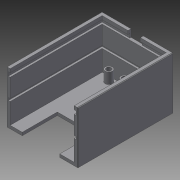
# Autodesk Inventor part: TOP
Saved by Autodesk Inventor 2014 SP1 (Build 180222100, 222)
## iProperties
Created: 2013-12-02
Part Number: TOP
Material: Generic
Document SubType Name: Modeling
Designer: Dominik
Density: 1 g/cm^3
Appearance: Default
Author: Dominik
Autodesk Inventor part; units mm, degrees
ref_plane "YZ Plane" through (0, 0, 0) normal (1, 0, 0) x (0, 1, 0)
ref_plane "XZ Plane" through (0, 0, 0) normal (0, 1, 0) x (-1, 0, 0)
ref_plane "XY Plane" through (0, 0, 0) normal (0, 0, 1) x (1, 0, 0)
sketch "Sketch1" plane through (0, 0, 0) normal (0, 0, 1) x (1, 0, 0)
  line L0 (0, 0) -> (59, 0)
  line L1 (59, 0) -> (59, 79)
  line L2 (59, 79) -> (0, 79)
  line L3 (0, 79) -> (0, 0)
  dimension "d0" = 59
  dimension "d1" = 79
  constraints: 8 end point, 1 horizontal, 1 vertical
  measures "d0" distance between parallel lines of L1 L3
  measures "d1" distance between parallel lines of L2 L0
extrude "Extrusion1" add sketch "Sketch1" along normal blind 3
sketch "Sketch2" plane through (0, 0, 3) normal (0, 0, 1) x (1, 0, 0)
  line L0 (59, 0) -> (59, 79) projected
  line L1 (0, 79) -> (0, 0) projected
  line L2 (0, 0) -> (0, 79) projected
  line L3 (0, 79) -> (59, 79) projected
  line L4 (59, 79) -> (59, 0) projected
  line L5 (59, 0) -> (0, 0) projected
  line L6 (3, 0) -> (56, 0)
  line L7 (56, 0) -> (56, 76)
  line L8 (56, 76) -> (3, 76)
  line L9 (3, 76) -> (3, 0)
  dimension "d25" = 3
  dimension "d26" = 3
  dimension "d27" = 3
  constraints: 8 end point, 1 point on line
  measures "d25" distance between parallel lines of L3 L8
  measures "d26" distance between parallel lines of L0 L7
  measures "d27" distance between parallel lines of L1 L9
extrude "Extrusion2" add sketch "Sketch2" along normal blind 40.5 contours L5 L7 L8 L9 L1 L3 L0
sketch "Sketch3" plane through (0, 0, 0) normal (0, 0, -1) x (-1, 0, 0)
  line L0 (0, 0) -> (-59, 0) projected
  line L1 (0, 79) -> (0, 0) projected
  line L2 (-59, 79) -> (0, 79) projected
  line L3 (-59, 0) -> (-59, 79) projected
  line L4 (-3, 76) -> (-3, 3) construction
  line L5 (-3, 3) -> (-56, 3) construction
  line L6 (-56, 3) -> (-56, 76) construction
  line L7 (-56, 76) -> (-3, 76) construction
  line L8 (-3, 76) -> (-56, 76) construction
  line L9 (-56, 76) -> (-56, 75) construction
  line L10 (-56, 75) -> (-3, 75) construction
  line L11 (-3, 75) -> (-3, 76) construction
  line L12 (-3, 75) -> (-9.5, 75) construction
  line L13 (-9.5, 75) -> (-9.5, 69) construction
  line L14 (-9.5, 69) -> (-3, 69) construction
  line L15 (-3, 69) -> (-3, 75) construction
  line L16 (-9.5, 69) -> (-15.5, 69) construction
  line L17 (-15.5, 69) -> (-15.5, 75) construction
  line L18 (-15.5, 75) -> (-9.5, 75) construction
  line L19 (-9.5, 75) -> (-9.5, 69) construction
  line L20 (-3, 69) -> (-22.5, 69) construction
  line L21 (-22.5, 69) -> (-22.5, 75) construction
  line L22 (-22.5, 75) -> (-3, 75) construction
  line L23 (-3, 75) -> (-3, 69) construction
  line L24 (-22.5, 69) -> (-28.5, 69) construction
  line L25 (-28.5, 69) -> (-28.5, 75) construction
  line L26 (-28.5, 75) -> (-22.5, 75) construction
  line L27 (-22.5, 75) -> (-22.5, 69) construction
  line L28 (-3, 69) -> (-35.5, 69) construction
  line L29 (-35.5, 69) -> (-35.5, 75) construction
  line L30 (-35.5, 75) -> (-3, 75) construction
  line L31 (-3, 75) -> (-3, 69) construction
  line L32 (-35.5, 69) -> (-41.5, 69) construction
  line L33 (-41.5, 69) -> (-41.5, 75) construction
  line L34 (-41.5, 75) -> (-35.5, 75) construction
  line L35 (-35.5, 75) -> (-35.5, 69) construction
  line L36 (-9.5, 69) -> (-15.5, 75) construction
  line L37 (-15.5, 69) -> (-9.5, 75) construction
  line L38 (-22.5, 69) -> (-28.5, 75) construction
  line L39 (-28.5, 69) -> (-22.5, 75) construction
  line L40 (-35.5, 69) -> (-41.5, 75) construction
  line L41 (-41.5, 69) -> (-35.5, 75) construction
  circle A0 centre (-12.5, 72) radius 3
  circle A1 centre (-25.5, 72) radius 3
  circle A2 centre (-38.5, 72) radius 3
  circle A3 centre (-12.5, 72) radius 2
  circle A4 centre (-25.5, 72) radius 2
  circle A5 centre (-38.5, 72) radius 2
  dimension "d9" = 3
  dimension "d10" = 1
  dimension "d11" = 6.5
  dimension "d12" = 6
  dimension "d13" = 6
  dimension "d14" = 19.5
  dimension "d15" = 6
  dimension "d16" = 32.5
  dimension "d17" = 6
  dimension "d18" = 1
  dimension "d19" = 1
  dimension "d20" = 1
  constraints: 76 end point, 6 centre point, 6 point on line, 5 horizontal, 5 vertical, 4 tangent, 3 coincident, 3 midpoint, 3 other
  measures "d9" distance between parallel lines of L2 L7
  measures "d10" distance between parallel lines of L8 L10
  measures "d11" distance between parallel lines of L15 L13
  measures "d12" distance between parallel lines of L12 L14
  measures "d13" distance between parallel lines of L17 L19
  measures "d14" distance between parallel lines of L21 L23
  measures "d15" distance between parallel lines of L25 L27
  measures "d16" distance between parallel lines of L29 L31
  measures "d17" distance between parallel lines of L33 L35
  measures "d18" radial gap between concentric circles of A0 A3
  measures "d19" radial gap between concentric circles of A1 A4
  measures "d20" radial gap between concentric circles of A2 A5
extrude "Extrusion3" add sketch "Sketch3" against normal blind 12 contours A0 | A1 | A2
sketch "Sketch4" plane through (12.5, 72, 3) normal (0, 0, 1) x (1, 0, 0)
  circle A0 centre (0, 0) radius 2 projected
  circle A1 centre (0, 0) radius 2
  circle A2 centre (26, 0) radius 2 projected
  circle A3 centre (26, 0) radius 3 projected
  circle A4 centre (0, 0) radius 2 projected
  circle A5 centre (0, 0) radius 3 projected
  circle A6 centre (13, 0) radius 2 projected
  circle A7 centre (13, 0) radius 3 projected
  circle A8 centre (13, 0) radius 2
  circle A9 centre (26, 0) radius 2
  line L0 (-12.5, -72) -> (-12.5, 7) projected
  line L1 (-12.5, 7) -> (46.5, 7) projected
  line L2 (46.5, 7) -> (46.5, -72) projected
  line L3 (46.5, -72) -> (43.5, -72) projected
  line L4 (43.5, -72) -> (-9.5, -72) projected
  line L5 (-9.5, -72) -> (-12.5, -72) projected
  line L6 (43.5, -72) -> (43.5, 4) projected
  line L7 (43.5, 4) -> (-9.5, 4) projected
  line L8 (-9.5, 4) -> (-9.5, -72) projected
  constraints: 3 centre point, 3 coincident
extrude "Extrusion4" cut sketch "Sketch4" against normal up to next contours A0 | A2 | A6
sketch "Sketch5" plane through (56, 0, 3) normal (-1, 0, 0) x (0, 0, 1)
  line L0 (40.5, 0) -> (0, 0) projected
  line L1 (0, 76) -> (40.5, 76) projected
  line L2 (0, 76) -> (17, 76) construction
  line L3 (17, 76) -> (17, 0) construction
  line L4 (17, 0) -> (0, 0) construction
  line L5 (0, 0) -> (0, 76) construction
  line L6 (17, 0) -> (19.2, 0)
  line L7 (19.2, 0) -> (19.2, 76)
  line L8 (19.2, 76) -> (17, 76)
  line L9 (17, 76) -> (17, 0)
  point P0 (-3, 0)
  dimension "d28" = 17
  dimension "d29" = 2.2
  constraints: 16 end point, 2 point on line
  measures "d28" distance between parallel lines of L5 L3
  measures "d29" distance between parallel lines of L9 L7
extrude "Extrusion5" cut sketch "Sketch5" against normal blind 1.5
sketch "Sketch8" plane through (3, 76, 3) normal (0, -1, 0) x (1, 0, 0)
  line L0 (0, 0) -> (0, 40.5) projected
  line L1 (54.5, 19.2) -> (0, 19.2)
  line L2 (0, 19.2) -> (0, 17)
  line L3 (0, 17) -> (54.5, 17)
  line L4 (54.5, 17) -> (54.5, 19.2)
  point P0 (-3, -3)
  constraints: 8 end point, 1 point on line
extrude "Extrusion8" cut sketch "Sketch8" against normal blind 1.5
sketch "Sketch9" plane through (3, 0, 3) normal (1, 0, 0) x (0, 0, -1)
  line L0 (0, 0) -> (-40.5, 0) projected
  line L1 (-19.2, 77.5) -> (-17, 77.5)
  line L2 (-17, 77.5) -> (-17, 0)
  line L3 (-17, 0) -> (-19.2, 0)
  line L4 (-19.2, 0) -> (-19.2, 77.5)
  point P0 (3, 0)
  constraints: 8 end point, 1 point on line
extrude "Extrusion9" cut sketch "Sketch9" against normal blind 1.5
sketch "Sketch10" plane through (56, 0, 43.5) normal (-1, 0, 0) x (0, 0, 1)
  line L0 (0, 0) -> (-21.3, 0) projected
  line L1 (-21.3, 76) -> (0, 76) projected
  line L2 (0, 0) -> (-2.9, 0) construction
  line L3 (-2.9, 0) -> (-2.9, 76) construction
  line L4 (-2.9, 76) -> (0, 76) construction
  line L5 (0, 76) -> (0, 0) construction
  line L6 (-2.9, 76) -> (-6.1, 76)
  line L7 (-6.1, 76) -> (-6.1, 0)
  line L8 (-6.1, 0) -> (-2.9, 0)
  line L9 (-2.9, 0) -> (-2.9, 76)
  point P0 (-43.5, 0)
  dimension "d40" = 2.9
  dimension "d41" = 3.2
  constraints: 16 end point, 2 point on line
  measures "d40" distance between parallel lines of L3 L5
  measures "d41" distance between parallel lines of L7 L9
extrude "Extrusion10" cut sketch "Sketch10" against normal blind 1.5
sketch "Sketch11" plane through (3, 76, 43.5) normal (0, -1, 0) x (1, 0, 0)
  line L0 (0, -21.3) -> (0, 0) projected
  line L1 (54.5, -2.9) -> (0, -2.9)
  line L2 (0, -2.9) -> (0, -6.1)
  line L3 (0, -6.1) -> (54.5, -6.1)
  line L4 (54.5, -6.1) -> (54.5, -2.9)
  point P0 (-3, -43.5)
  constraints: 8 end point, 1 point on line
extrude "Extrusion11" cut sketch "Sketch11" against normal blind 1.5
sketch "Sketch12" plane through (3, 0, 43.5) normal (1, 0, 0) x (0, 0, -1)
  line L0 (21.3, 0) -> (0, 0) projected
  line L1 (6.1, 77.5) -> (2.9, 77.5)
  line L2 (2.9, 77.5) -> (2.9, 0)
  line L3 (2.9, 0) -> (6.1, 0)
  line L4 (6.1, 0) -> (6.1, 77.5)
  point P0 (43.5, 0)
  constraints: 8 end point, 1 point on line
extrude "Extrusion12" cut sketch "Sketch12" against normal blind 1.5
sketch "Sketch13" plane through (0, 0, 43.5) normal (0, 0, 1) x (1, 0, 0)
  line L0 (3, 76) -> (56, 76) projected
  line L1 (59, 0) -> (59, 79) projected
  line L2 (59, 79) -> (0, 79) projected
  line L3 (0, 79) -> (24.4, 79) construction
  line L4 (24.4, 79) -> (24.4, 76) construction
  line L5 (24.4, 76) -> (0, 76) construction
  line L6 (0, 76) -> (0, 79) construction
  line L7 (34.6, 79) -> (59, 79) construction
  line L8 (59, 79) -> (59, 76) construction
  line L9 (59, 76) -> (34.6, 76) construction
  line L10 (34.6, 76) -> (34.6, 79) construction
  line L11 (24.4, 79) -> (34.6, 79)
  line L12 (34.6, 79) -> (34.6, 76)
  line L13 (34.6, 76) -> (24.4, 76)
  line L14 (24.4, 76) -> (24.4, 79)
  dimension "d48" = 24.4
  dimension "d49" = 24.4
  dimension "d50" = 10.2
  constraints: 24 end point, 3 point on line
  measures "d48" distance between parallel lines of L6 L4
  measures "d49" distance between parallel lines of L1 L10
  measures "d50" distance between parallel lines of L10 L4
extrude "Extrusion13" cut sketch "Sketch13" against normal blind 6.1
sketch "Sketch14" plane through (0, 0, 3) normal (0, 0, 1) x (1, 0, 0)
  line L0 (56, 0) -> (56, 76) projected
  line L1 (3, 76) -> (3, 0) projected
  line L2 (3, 0) -> (56, 0) projected
  line L3 (3, 0) -> (13, 0) construction
  line L4 (13, 0) -> (13, 29) construction
  line L5 (13, 29) -> (3, 29) construction
  line L6 (3, 29) -> (3, 0) construction
  line L7 (13, 29) -> (44, 29)
  line L8 (44, 29) -> (44, 0)
  line L9 (44, 0) -> (13, 0)
  line L10 (13, 0) -> (13, 29)
  point P0 (0, 0)
  dimension "d53" = 29
  dimension "d54" = 10
  dimension "d55" = 12
  constraints: 16 end point, 1 point on line
  measures "d53" distance between parallel lines of L3 L5
  measures "d54" distance between parallel lines of L1 L4
  measures "d55" distance between parallel lines of L0 L8
extrude "Extrusion14" cut sketch "Sketch14" against normal up to next
chamfer "Chamfer1" distance 0.5 angle 45 19 edges at (46.8, 79, 43.5) (59, 39.5, 43.5) (12.2, 79, 43.5) (0, 39.5, 43.5) (0, 0, 21.75) (6.5, 0, 0) (51.5, 0, 0) (59, 0, 21.75) (59, 39.5, 0) (0, 39.5, 0) (29.5, 79, 0) (10.5, 72, 0) (23.5, 72, 0) (36.5, 72, 0) (59, 79, 21.75) (0, 79, 21.75) (24.4, 79, 40.45) (29.5, 79, 37.4) (34.6, 79, 40.45)
chamfer "Chamfer2" distance 0.5 angle 45 3 edges at (13, 14.75, 0) (28.5, 29, 0) (44, 14.75, 0)
equation "\"d26\" = d25"
equation "\"d27\" = d26"
equation "\"d20\" = d19"
equation "\"d49\" = d48"
body "Solid1"
